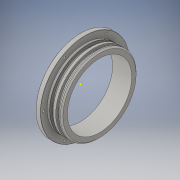
# Autodesk Inventor part: THE ACTUAL O-RONG FITTING, CORRECT DIMENSIONS
Saved by Autodesk Inventor 2016 (Build 200138000, 138)
## iProperties
Created: 2017-03-06
Part Number: THE ACTUAL O-RONG FITTING, CORRECT DIMENSIONS
Material: Generic
Document SubType Name: Modeling
Designer: Student
Density: 1 g/cm^3
Appearance: Default
Author: Student
Autodesk Inventor part; units mm, degrees
ref_plane "YZ Plane" through (0, 0, 0) normal (1, 0, 0) x (0, 1, 0)
ref_plane "XZ Plane" through (0, 0, 0) normal (0, 1, 0) x (-1, 0, 0)
ref_plane "XY Plane" through (0, 0, 0) normal (0, 0, 1) x (1, 0, 0)
sketch "Sketch1" plane through (0, 0, 0) normal (0, 1, 0) x (-1, 0, 0)
  line L0 (-0.762, -0.635) -> (2.667, -0.635)
  line L1 (-0.762, -0.635) -> (-0.762, -4.445)
  line L2 (-0.762, -4.445) -> (-5.207, -4.445)
  line L3 (-5.207, -4.445) -> (-5.207, -0.635)
  line L4 (-5.207, -0.635) -> (-8.763, -0.635)
  line L5 (-8.763, -0.635) -> (-8.763, -4.445)
  line L6 (-8.763, -4.445) -> (-13.208, -4.445)
  line L7 (-13.208, -4.445) -> (-13.208, -0.635)
  line L8 (-13.208, -0.635) -> (-16.51, -0.635)
  line L9 (-16.51, -0.635) -> (-16.51, -8.255)
  line L10 (-16.51, -8.255) -> (2.667, -8.255)
  line L11 (2.667, -8.255) -> (2.667, -0.635)
  line L12 (-15.24, -50.927) -> (-2.54, -50.927) construction
  line L13 (-6.0325, 0) -> (-6.0325, -1.397) construction
  line L14 (-14.859, -0.635) -> (-14.859, -5.1188) construction
  line L15 (2.2225, 0) -> (2.2225, -1.397) construction
  line L16 (-15.24, -8.255) -> (-15.24, -50.927) construction
  dimension "d2" = 4.445
  dimension "d3" = 3.556
  dimension "d4" = 4.445
  dimension "d5" = 3.302
  dimension "d38" = 12.7
  dimension "d65" = 3.81
  dimension "d66" = 3.81
  dimension "d67" = 3.81
  dimension "d68" = 1.397
  dimension "d71" = 19.177
  dimension "d72" = 42.672
  dimension "d73" = 7.62
  dimension "d74" = 7.62
  constraints: 34 end point, 7 perpendicular, 5 vertical, 2 horizontal, 2 point on line, 1 midpoint
  measures "d2" distance of L1.end L2.end
  measures "d3" distance of L3.end L4.end
  measures "d4" distance of L5.end L6.end
  measures "d5" distance of L7.end L8.end
  measures "d38" distance of L12.start L12.end
  measures "d65" distance from line of L14.start L6
  measures "d66" distance between parallel lines of L4 L6
  measures "d67" distance between parallel lines of L0 L2
  measures "d68" distance of L13.start L13.end
  measures "d71" distance of L9.end L10.end
  measures "d72" distance of L16.start L12.start
  measures "d73" distance of L8.end L9.end
  measures "d74" distance of L10.end L0.end
revolve "Revolution1" add sketch "Sketch1" angle 360 about axis through (15.24, 0, -50.927) along (-1, 0, 0)
sketch "Sketch2" plane through (-2.667, 0, -50.927) normal (-1, 0, 0) x (0, 0, 1)
  circle A0 centre (0, 0) radius 59.055
  circle A1 centre (0, 0) radius 42.672 projected
  dimension "d10" = 118.11
  constraints: 1 centre point, 1 coincident
  measures "d10" diameter of A0
extrude "Extrusion1" add sketch "Sketch2" along normal blind 6.096
sketch "Sketch3" plane through (-8.763, 0, -50.927) normal (-1, 0, 0) x (0, 0, 1)
  circle A0 centre (0, 0) radius 48.5013
  circle A1 centre (0, 0) radius 51.6763
  circle A2 centre (0, 0) radius 42.672 construction
  dimension "d42" = 3.175
  dimension "d62" = 97.0026
  constraints: 2 centre point, 2 coincident
  measures "d42" radial gap between concentric circles of A1 A0
  measures "d62" diameter of A0
extrude "Extrusion2" cut sketch "Sketch3" against normal blind 3.5306
chamfer "Chamfer1" distance 1.778 angle 45 1 edges at (16.51, 0, -101.219)
sketch "Sketch5" plane through (-8.763, 0, -50.927) normal (-1, 0, 0) x (0, 0, 1)
  circle A0 centre (0, 0) radius 55.245 construction
  circle A1 centre (0, 0) radius 42.672 projected
  circle A2 centre (0, 0) radius 48.5013 projected
  point P0 (-55.245, 0)
  point P1 (-27.6225, -47.8436)
  point P2 (27.6225, -47.8436)
  point P3 (55.245, 0)
  point P4 (27.6225, 47.8436)
  point P5 (-27.6225, 47.8436)
  dimension "d43" = 110.49
  dimension "d46" = 360
  constraints: 2 horizontal alignment, 10 other
hole "Hole1" at (-8.763, 0, -106.172) at (-8.763, -47.8436, -78.5495) at (-8.763, -47.8436, -23.3045) at (-8.763, 0, 4.318) at (-8.763, 47.8436, -23.3045) at (-8.763, 47.8436, -78.5495) direction (1, 0, 0) diameter 3 end through all
chamfer "Chamfer2" distance 0.254 angle 45 5 edges at (0.762, 0, -101.219) (-8.763, 0, -102.6033) (-8.763, 0, -99.4283) (-8.763, 0, -109.982) (-2.667, 0, -109.982)
sketch "Sketch8" plane through (-8.763, 0, -50.927) normal (-1, 0, 0) x (0, 0, 1)
  circle A0 centre (0, 0) radius 48.2473 projected
  point P0 (50.927, 0)
equation "\"d66\" = d65"
equation "\"d67\" = d66"
body "Solid1"
